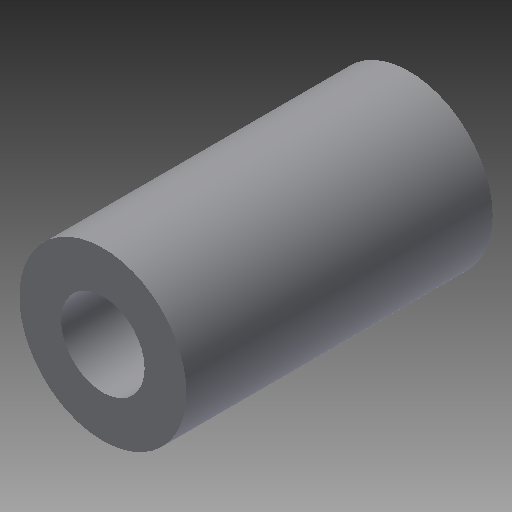
# Autodesk Inventor part: Kupplung
Saved by Autodesk Inventor 2018 (Build 220112000, 112)
## iProperties
Created: 2013-02-20
Part Number: Kupplung
Material: Generic
Document SubType Name: Modeling
Designer: Neef
Density: 1 g/cm^3
Appearance: Default
Author: Neef
Autodesk Inventor part; units mm, degrees
ref_plane "YZ Plane" through (0, 0, 0) normal (1, 0, 0) x (0, 1, 0)
ref_plane "XZ Plane" through (0, 0, 0) normal (0, 1, 0) x (-1, 0, 0)
ref_plane "XY Plane" through (0, 0, 0) normal (0, 0, 1) x (1, 0, 0)
sketch "Skizze1" plane through (0, 0, 0) normal (0, 0, 1) x (1, 0, 0)
  line L0 (0, 4.4) -> (0, -26.4) projected
  line L1 (-1.2, 0) -> (7.2, 0) projected
  line L2 (2.25, 0) -> (6, 0)
  line L3 (6, 0) -> (6, -22)
  line L4 (6, -22) -> (3, -22)
  line L5 (2.25, -11) -> (2.25, 0)
  line L6 (2.25, -11) -> (3, -11)
  line L7 (3, -11) -> (3, -22)
  point P0 (0, 0)
  dimension "d0" = 22
  dimension "d1" = 6
  dimension "d2" = 3
  dimension "d3" = 11
  dimension "d4" = 2.25
  constraints: 12 end point, 3 perpendicular, 2 parallel, 1 horizontal, 1 point on line
  measures "d0" distance of L2.end L3.end
  measures "d1" distance between parallel lines of L0 L3
  measures "d2" distance between parallel lines of L0 L7
  measures "d3" distance of L6.end L4.end
  measures "d4" distance between parallel lines of L0 L5
revolve "Umdrehung1" add sketch "Skizze1" angle 360 about axis through (0, 0, 0) along (0, -1, 0)
equation "\"d3\" = 0.5 * d0"
